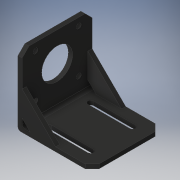
# Autodesk Inventor part: Motor mount NEMA 17
Saved by Autodesk Inventor 2017 (Build 210142000, 142)
## iProperties
Part Number: Motor mount NEMA 17
Material: Stahl, unlegiert
Document SubType Name: Modeling
Designer: Till
Density: 7.85 g/cm^3
Appearance: Eisen schwarz
Author: Till
Autodesk Inventor part; units mm, degrees
ref_plane "YZ Plane" through (0, 0, 0) normal (1, 0, 0) x (0, 1, 0)
ref_plane "XZ Plane" through (0, 0, 0) normal (0, 1, 0) x (-1, 0, 0)
ref_plane "XY Plane" through (0, 0, 0) normal (0, 0, 1) x (1, 0, 0)
sketch "Skizze1" plane through (0, 0, 0) normal (0, 0, 1) x (1, 0, 0)
  line L0 (0, 0) -> (0, 50)
  line L1 (0, 50) -> (48, 50)
  line L2 (53, 45) -> (53, 5)
  line L3 (48, 0) -> (0, 0)
  line L4 (12, 40) -> (42, 40) construction
  line L5 (12, 37.9) -> (42, 37.9)
  line L6 (42, 42.1) -> (12, 42.1)
  arc A0 (12, 42.1) -> (12, 37.9) centre (12, 40) ccw
  arc A1 (42, 37.9) -> (42, 42.1) centre (42, 40) ccw
  line L7 (12, 10) -> (42, 10) construction
  line L8 (12, 7.9) -> (42, 7.9)
  line L9 (42, 12.1) -> (12, 12.1)
  arc A2 (12, 12.1) -> (12, 7.9) centre (12, 10) ccw
  arc A3 (42, 7.9) -> (42, 12.1) centre (42, 10) ccw
  line L10 (48, 50) -> (53, 45)
  line L11 (53, 5) -> (48, 0)
  point P0 (53, 50)
  point P1 (53, 0)
  point P2 (27, 40)
  point P3 (27, 10)
  dimension "d0" = 50
  dimension "d1" = 53
  dimension "d2" = 30
  dimension "d3" = 4.2
  dimension "d4" = 10
  dimension "d5" = 11
  dimension "d6" = 4.2
  dimension "d7" = 10
  dimension "d8" = 11
  dimension "d9" = 5
  dimension "d10" = 5
  dimension "d11" = 5
  dimension "d12" = 5
  constraints: 28 end point, 8 point on circle, 8 tangent, 4 centre point, 4 point on line, 3 perpendicular, 2 horizontal, 2 midpoint, 2 parallel, 1 vertical
  measures "d0" distance of L0.start L0.end
  measures "d1" distance of L0.end point (53, 50)
  measures "d2" distance of L4.start L4.end
  measures "d3" diameter of A1
  measures "d4" distance from line of L1 point (27, 40)
  measures "d5" distance from line of L2 L4.end
  measures "d6" diameter of A3
  measures "d7" distance from line of L3 point (27, 10)
  measures "d8" distance from line of L2 L7.end
  measures "d9" distance of L1.end point (53, 50)
  measures "d10" distance of L2.start point (53, 50)
  measures "d11" distance of L2.end point (53, 0)
  measures "d12" distance of L3.start point (53, 0)
extrude "Extrusion1" add sketch "Skizze1" along normal blind 3
sketch "Skizze2" plane through (0, 0, 0) normal (-1, 0, 0) x (0, 0, 1)
  line L0 (0, 50) -> (3, 50) projected
  line L1 (0, 50) -> (46, 50)
  line L2 (51, 45) -> (51, 5)
  line L3 (46, 0) -> (0, 0)
  line L4 (0, 0) -> (0, 50)
  line L5 (46, 50) -> (51, 45)
  line L6 (51, 5) -> (46, 0)
  circle A0 centre (30, 25) radius 11.05
  circle A1 centre (45.6319, 40.5) radius 1.75
  circle A2 centre (45.6319, 9.5) radius 1.75
  circle A3 centre (14.6319, 9.5) radius 1.75
  circle A4 centre (14.6319, 40.5) radius 1.75
  line L7 (30.1319, 50) -> (30.1319, 0) construction
  line L8 (51, 25) -> (0, 25) construction
  point P0 (51, 0)
  point P1 (51, 50)
  dimension "d15" = 51
  dimension "d16" = 5
  dimension "d17" = 5
  dimension "d18" = 5
  dimension "d19" = 5
  dimension "d20" = 22.1
  dimension "d21" = 3.5
  dimension "d22" = 21
  dimension "d23" = 3.5
  dimension "d24" = 3.5
  dimension "d25" = 3.5
  dimension "d26" = 31
  dimension "d27" = 31
  dimension "d28" = 31
  dimension "d29" = 31
  dimension "d30" = 15.5
  dimension "d31" = 15.5
  dimension "d32" = 15.5
  dimension "d33" = 15.5
  constraints: 16 end point, 6 point on line, 5 centre point, 2 midpoint, 2 parallel, 2 perpendicular, 1 horizontal
  measures "d15" distance of point (51, 0) L3.end
  measures "d16" distance of L1.end point (51, 50)
  measures "d17" distance of L2.start point (51, 50)
  measures "d18" distance of L2.end point (51, 0)
  measures "d19" distance of L3.start point (51, 0)
  measures "d20" diameter of A0
  measures "d21" diameter of A1
  measures "d22" distance from line of L2 A0.centre
  measures "d23" diameter of A2
  measures "d24" diameter of A3
  measures "d25" diameter of A4
  measures "d26" distance of A2.centre A1.centre
  measures "d27" distance of A3.centre A2.centre
  measures "d28" distance of A4.centre A1.centre
  measures "d29" distance of A3.centre A4.centre
  measures "d30" distance from line of L7 A1.centre
  measures "d31" distance from line of L8 A1.centre
  measures "d32" distance from line of L8 A2.centre
  measures "d33" distance from line of L8 A3.centre
extrude "Extrusion2" add sketch "Skizze2" against normal blind 3
sketch "Skizze3" plane through (0, 0, 0) normal (0, -1, 0) x (1, 0, 0)
  line L0 (3, 3) -> (48, 3) projected
  line L1 (8.8368, 3) -> (3, 8.8368)
  line L2 (8.8368, 3) -> (17.0913, 3) construction
  line L3 (3, 8.8368) -> (3, 26.8368)
  line L4 (3, 46) -> (3, 3) projected
  line L5 (3, 26.8368) -> (26.8368, 3)
  line L6 (42, 3) -> (12, 3) projected
  line L7 (26.8368, 3) -> (8.8368, 3)
  point P0 (0, 0)
  dimension "d36" = 135
  dimension "d37" = 18
  dimension "d38" = 45
  constraints: 10 end point, 3 point on line, 1 equal length, 1 horizontal, 1 perpendicular
  measures "d36" angle of L2 L1
  measures "d37" distance of L1.end L3.end
  measures "d38" angle of L3 L5
extrude "Extrusion3" add sketch "Skizze3" against normal blind 3 contours L1 L3 L5 L0
sketch "Skizze4" plane through (0, 50, 0) normal (0, 1, 0) x (1, 0, 0)
  line L0 (42, -3) -> (12, -3) projected
  line L1 (3, -46) -> (3, -26.8368) projected
  line L2 (27, -3) -> (3, -26.8368)
  line L3 (8.8368, -3) -> (3, -8.8368) projected
  line L4 (3, -26.8368) -> (3, -8.8368)
  line L5 (3, -8.8368) -> (8.8368, -3)
  line L6 (8.8368, -3) -> (27, -3)
  point P0 (0, 0)
  constraints: 8 end point, 1 collinear, 1 midpoint, 1 perpendicular, 1 vertical
extrude "Extrusion4" add sketch "Skizze4" against normal blind 3
fillet "Rundung1" radius 2 2 edges at (0, 25, 0) (3, 25, 3)
equation "\"d12\" = d11"
equation "\"d17\" = d16"
equation "\"d18\" = d16"
equation "\"d19\" = d18"
